Autodesk Inventor part; units mm, degrees
(part 2 of 2)
  spline S321 degree 2 poles (3.6258, 20.9215) (3.6199, 20.9948) (3.5664, 21.0859) (3.5327, 21.0859) knots 0 0 0 1 2 2 2
  spline S322 degree 2 poles (3.5327, 21.0859) (3.499, 21.0859) (3.4634, 20.9294) (3.4574, 20.7491) knots 0 0 0 1 2 2 2
  line L277 (3.4574, 20.7491) -> (3.4039, 20.7491)
  spline S323 degree 2 poles (3.4039, 20.7491) (3.4, 21.0206) (3.4792, 21.3475) (3.5426, 21.3475) knots 0 0 0 1 2 2 2
  spline S324 degree 2 poles (3.5426, 21.3475) (3.6041, 21.3475) (3.6892, 21.1315) (3.6892, 20.979) knots 0 0 0 1 2 2 2
  line L278 (3.6892, 20.979) -> (3.6892, 19.7426)
  spline S325 degree 2 poles (3.6892, 19.7426) (3.6892, 19.705) (3.7031, 19.6436) (3.713, 19.6356) knots 0 0 0 1 2 2 2
  spline S326 degree 2 poles (3.713, 19.6356) (3.719, 19.6317) (3.7289, 19.6356) knots 0 0 0 1 1 1
  line L279 (3.7289, 19.6356) -> (3.7289, 19.4177)
  line L280 (3.6278, 20.0715) -> (3.6278, 20.3549)
  spline S327 degree 2 poles (3.6278, 20.3549) (3.5842, 20.2954) (3.501, 20.234) knots 0 0 0 1 1 1
  spline S328 degree 2 poles (3.501, 20.234) (3.4792, 20.2122) (3.4475, 20.0378) (3.4475, 19.9289) knots 0 0 0 1 2 2 2
  spline S329 degree 2 poles (3.4475, 19.9289) (3.4475, 19.8041) (3.4852, 19.6356) (3.5129, 19.6356) knots 0 0 0 1 2 2 2
  spline S330 degree 2 poles (3.5129, 19.6356) (3.5605, 19.6356) (3.6278, 19.9011) (3.6278, 20.0715) knots 0 0 0 1 2 2 2
  spline S331 degree 2 poles (3.9211, 19.4078) (3.8953, 19.384) (3.8715, 19.384) knots 0 0 0 1 1 1
  spline S332 degree 2 poles (3.8715, 19.384) (3.8418, 19.384) (3.822, 19.4712) knots 0 0 0 1 1 1
  spline S333 degree 2 poles (3.822, 19.4712) (3.8061, 19.5485) (3.8061, 19.6495) knots 0 0 0 1 1 1
  line L281 (3.8061, 19.6495) -> (3.8061, 21.0285)
  line L282 (3.8061, 21.0285) -> (3.7546, 21.0285)
  line L283 (3.7546, 21.0285) -> (3.7546, 21.296)
  line L284 (3.7546, 21.296) -> (3.8061, 21.296)
  line L285 (3.8061, 21.296) -> (3.8061, 21.7913)
  line L286 (3.8061, 21.7913) -> (3.8656, 21.7913)
  line L287 (3.8656, 21.7913) -> (3.8656, 21.296)
  line L288 (3.8656, 21.296) -> (3.9211, 21.296)
  line L289 (3.9211, 21.296) -> (3.9211, 21.0285)
  line L290 (3.9211, 21.0285) -> (3.8656, 21.0285)
  line L291 (3.8656, 21.0285) -> (3.8656, 19.7387)
  spline S334 degree 2 poles (3.8656, 19.7387) (3.8656, 19.6515) (3.8894, 19.6515) knots 0 0 0 1 1 1
  spline S335 degree 2 poles (3.8894, 19.6515) (3.9012, 19.6515) (3.9211, 19.6693) knots 0 0 0 1 1 1
  line L292 (3.9211, 19.6693) -> (3.9211, 19.4078)
  line L293 (4.2381, 19.4672) -> (4.1786, 19.4672)
  line L294 (4.1786, 19.4672) -> (4.1786, 21.296)
  line L295 (4.1786, 21.296) -> (4.2381, 21.296)
  line L296 (4.2381, 21.296) -> (4.2381, 19.4672)
  line L297 (4.2381, 21.6447) -> (4.1786, 21.6447)
  line L298 (4.1786, 21.6447) -> (4.1786, 22.0072)
  line L299 (4.1786, 22.0072) -> (4.2381, 22.0072)
  line L300 (4.2381, 22.0072) -> (4.2381, 21.6447)
  spline S336 degree 2 poles (4.4639, 19.4078) (4.4382, 19.384) (4.4144, 19.384) knots 0 0 0 1 1 1
  spline S337 degree 2 poles (4.4144, 19.384) (4.3847, 19.384) (4.3649, 19.4712) knots 0 0 0 1 1 1
  spline S338 degree 2 poles (4.3649, 19.4712) (4.349, 19.5485) (4.349, 19.6495) knots 0 0 0 1 1 1
  line L301 (4.349, 19.6495) -> (4.349, 21.0285)
  line L302 (4.349, 21.0285) -> (4.2975, 21.0285)
  line L303 (4.2975, 21.0285) -> (4.2975, 21.296)
  line L304 (4.2975, 21.296) -> (4.349, 21.296)
  line L305 (4.349, 21.296) -> (4.349, 21.7913)
  line L306 (4.349, 21.7913) -> (4.4084, 21.7913)
  line L307 (4.4084, 21.7913) -> (4.4084, 21.296)
  line L308 (4.4084, 21.296) -> (4.4639, 21.296)
  line L309 (4.4639, 21.296) -> (4.4639, 21.0285)
  line L310 (4.4639, 21.0285) -> (4.4084, 21.0285)
  line L311 (4.4084, 21.0285) -> (4.4084, 19.7387)
  spline S339 degree 2 poles (4.4084, 19.7387) (4.4084, 19.6515) (4.4322, 19.6515) knots 0 0 0 1 1 1
  spline S340 degree 2 poles (4.4322, 19.6515) (4.4441, 19.6515) (4.4639, 19.6693) knots 0 0 0 1 1 1
  line L312 (4.4639, 19.6693) -> (4.4639, 19.4078)
  line L313 (4.6125, 19.4672) -> (4.5392, 19.4672)
  line L314 (4.5392, 19.4672) -> (4.5392, 19.8258)
  line L315 (4.5392, 19.8258) -> (4.6125, 19.8258)
  line L316 (4.6125, 19.8258) -> (4.6125, 19.4672)
  point P0 (3.6667, 35.56)
  constraints: 2 other
emboss "Emboss1" sketch "Sketch3" operation cut depth 2.54 direction (-0.000265, -1, 0)
body "Solid1"
